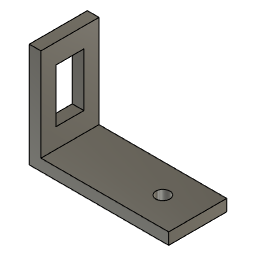
držač motora kamere (Autodesk Fusion 360 design; units mm, degrees)
Autodesk Fusion 360 part; units mm, degrees
sketch "Sketch1" plane through (0, 0, 0) normal (0, 0, 1) x (1, 0, 0)
  circle A0 centre (0, 0) radius 3
  line L0 (15, -12.5) -> (-45, -12.5)
  line L1 (-45, -12.5) -> (-45, 12.5)
  line L2 (-45, 12.5) -> (15, 12.5)
  line L3 (15, 12.5) -> (15, -12.5)
  dimension "d1" = 6
  dimension "d2" = 25
  dimension "d12" = 60
  dimension "d14" = 15
  constraint coincident A0.centre origin
  constraint horizontal L0
  constraint perpendicular L0 L1
  constraint parallel L0 L2
  constraint parallel L1 L3
  measures "d1" diameter of A0
  measures "d2" distance of L0.end L1.end
  measures "d12" distance of L1.end L2.end
  measures "d14" distance of A0.centre L3
extrude "Extrude1" add sketch "Sketch1" along normal blind 5
sketch "Sketch2" plane through (0, 0, 5) normal (0, 0, 1) x (-1, 0, 0)
  circle A0 centre (0, 0) radius 3
  line L0 (-15, -12.5) -> (45, -12.5)
  line L1 (45, -12.5) -> (45, 12.5)
  line L2 (45, 12.5) -> (-15, 12.5)
  line L3 (-15, 12.5) -> (-15, -12.5)
  line L4 (45, -12.5) -> (40, -12.5)
  line L5 (40, -12.5) -> (40, 12.5)
  line L6 (40, 12.5) -> (45, 12.5)
  line L7 (45, 12.5) -> (45, -12.5)
  dimension "d5" = 5
  constraint horizontal L4
  constraint vertical L5
  constraint horizontal L6
  constraint vertical L7
  constraint coincident L0.end L1.start
  measures "d5" distance of L0.end L4.end
extrude "Extrude2" add sketch "Sketch2" along normal blind 40 contours L0 L1 L2 L4 L5 L6 L7
sketch "Sketch3" plane through (-40, 0, 0) normal (1, 0, 0) x (0, 1, 0)
  line L0 (-12.5, 5) -> (12.5, 5)
  line L1 (12.5, 5) -> (12.5, 45)
  line L2 (12.5, 45) -> (-12.5, 45)
  line L3 (-12.5, 45) -> (-12.5, 5)
  line L4 (6, 13.5) -> (-6, 13.5)
  line L5 (-6, 13.5) -> (-6, 36.5)
  line L6 (-6, 36.5) -> (6, 36.5)
  line L7 (6, 36.5) -> (6, 13.5)
  line L8 (6, 13.5) -> (-6, 36.5) construction
  line L9 (-6, 13.5) -> (6, 36.5) construction
  point P0 (0, 25)
  dimension "d8" = 12
  dimension "d9" = 23
  constraint horizontal L4
  constraint perpendicular L4 L5
  constraint parallel L4 L6
  constraint parallel L5 L7
  constraint coincident L8 P0
  constraint coincident L9 P0
  measures "d8" distance of L5.end L6.end
  measures "d9" distance of L4.end L5.end
extrude "Extrude3" cut sketch "Sketch3" against normal blind 40 contours L4 L5 L6 L7
